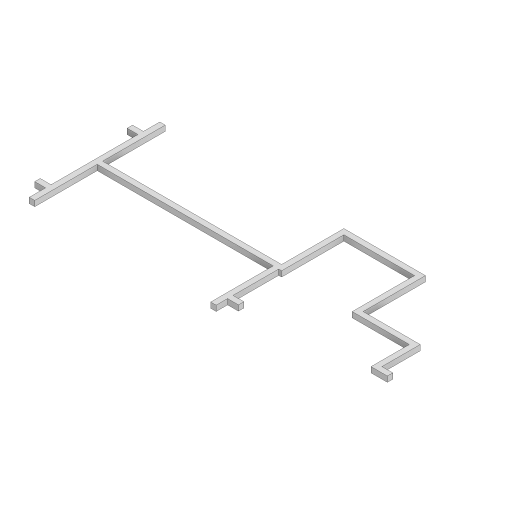
# Autodesk Inventor part: Positioning Stencil
Saved by Autodesk Inventor 2023.4 (Build 274418000, 418)
## iProperties
Created: 2024-03-21
Part Number: Positioning Stencil
Material: Generic
Document SubType Name: Modeling
Designer: josep
Density: 1 g/cm^3
Appearance: Default
Author: josep
Autodesk Inventor part; units mm, degrees
ref_plane "YZ Plane" through (0, 0, 0) normal (1, 0, 0) x (0, 1, 0)
ref_plane "XZ Plane" through (0, 0, 0) normal (0, 1, 0) x (-1, 0, 0)
ref_plane "XY Plane" through (0, 0, 0) normal (0, 0, 1) x (1, 0, 0)
sketch "Sketch1" plane through (0, 0, 0) normal (0, 1, 0) x (-1, 0, 0)
  line L0 (142.3035, 60) -> (-142.3035, 60)
  line L1 (-142.3035, 60) -> (-142.3035, -60)
  line L2 (-142.3035, -60) -> (142.3035, -60)
  line L3 (142.3035, -60) -> (142.3035, 60)
  line L4 (142.3035, 45) -> (122.3035, 45)
  line L5 (122.3035, 45) -> (122.3035, -45)
  line L6 (122.3035, -45) -> (142.3035, -45)
  line L7 (132.3035, 45) -> (132.3035, 40)
  line L8 (132.3035, 40) -> (122.3035, 40)
  line L9 (132.3035, -45) -> (132.3035, -40)
  line L10 (132.3035, -40) -> (122.3035, -40)
  line L11 (122.3035, -45) -> (122.3035, -60)
  line L12 (117.3035, -60) -> (117.3035, -2.5)
  line L13 (117.3035, -2.5) -> (-142.3035, -2.5)
  line L14 (122.3035, 45) -> (122.3035, 60)
  line L15 (117.3035, 60) -> (117.3035, 2.5)
  line L16 (117.3035, 2.5) -> (-142.3035, 2.5)
  line L17 (-169.8065, 2.5) -> (-169.8065, 37.7)
  line L18 (-169.8065, 37.7) -> (-142.3035, 37.7)
  line L19 (-142.3035, 32.7) -> (-174.8065, 32.7)
  line L20 (-174.8065, 32.7) -> (-174.8065, 2.5)
  line L21 (-49.5965, 60) -> (-49.5965, 67.5)
  line L22 (-49.5965, 60) -> (-49.5965, 67.5)
  line L23 (-49.5965, 60) -> (-49.5965, 55.5)
  line L24 (-44.5965, 49.5) -> (-49.5965, 49.5)
  line L25 (-49.5965, 49.5) -> (-49.5965, 55.5)
  line L26 (-44.5965, 29.5) -> (-44.5965, 2.5)
  line L27 (-49.5965, 50.5) -> (-49.5965, 2.5)
  line L28 (-47.3065, -2.5) -> (-47.3065, -39.629)
  line L29 (-117.3065, -39.629) -> (-117.3065, -35.2)
  line L30 (-52.3065, -35.2) -> (-52.3065, -2.5)
  line L31 (-174.8065, 2.5) -> (-174.8065, -2.5)
  line L32 (-117.3065, -35.2) -> (-117.3065, -2.5)
  line L33 (-122.3065, -2.5) -> (-122.3065, -39.629)
  line L34 (-122.3065, -39.629) -> (-117.3065, -39.629)
  line L35 (-117.3065, -2.5) -> (-117.3065, 2.5)
  line L36 (-122.3065, -2.5) -> (-122.3065, 2.5)
  line L37 (-52.3065, -2.5) -> (-52.3065, 2.5)
  line L38 (-47.3065, -39.629) -> (-47.3065, -59.8)
  line L39 (-47.3065, -59.8) -> (-52.3065, -59.8)
  line L40 (-52.3065, -59.8) -> (-52.3065, -35.2)
  line L41 (-52.3065, -59.8) -> (-122.3065, -59.8)
  line L42 (-122.3065, -59.8) -> (-122.3065, -39.629)
  line L43 (-117.3065, -39.629) -> (-117.3065, -59.8)
  line L44 (-52.3065, -54.8) -> (-117.3065, -54.8)
  line L45 (0, -2.5) -> (0, 2.5)
  line L46 (-174.8065, 32.7) -> (-184.8065, 32.7)
  line L47 (-184.8065, 32.7) -> (-184.8065, 37.7)
  line L48 (-184.8065, 37.7) -> (-142.3035, 37.7)
  line L49 (-44.5965, 29.5) -> (-44.5965, 49.5)
  line L50 (-49.5965, 49.9226) -> (-49.5965, 49.5)
  line L51 (-44.5965, 49.5) -> (-44.5965, 64.5)
  line L52 (-44.5965, 64.5) -> (-49.5965, 64.5)
  line L53 (-49.5965, 49.5) -> (-59.5965, 49.5)
  line L54 (-59.5965, 49.5) -> (-59.5965, 44.5)
  line L55 (-59.5965, 44.5) -> (-49.5965, 44.5)
  line L56 (117.3035, -2.5) -> (117.3035, 2.5)
  line L57 (-142.3035, -2.5) -> (-174.8065, -2.5)
  line L58 (-142.3035, 2.5) -> (-169.8065, 2.5)
  point P0 (0, 0)
  point P1 (142.3035, 0)
  point P2 (0, -60)
  point P3 (-158.555, 32.7)
  point P4 (-14.5965, 67.5)
  point P5 (-14.5965, 60)
  point P6 (-159.8035, 32.7)
  point P7 (-44.5965, 60)
  point P8 (-169.8065, 32.7)
  dimension "d0" = 284.607
  dimension "d1" = 120
  dimension "d2" = 15
  dimension "d3" = 15
  dimension "d4" = 10
  dimension "d5" = 5
  dimension "d6" = 5
  dimension "d7" = 5
  dimension "d14" = 0
  dimension "d15" = 0
  dimension "d17" = 12.3
  dimension "d18" = 57.5
  dimension "d19" = 57.5
  dimension "d20" = 5
  dimension "d26" = 171.9
  dimension "d30" = 4.5
  dimension "d34" = 20
  dimension "d36" = 174.61
  dimension "d37" = 5
  dimension "d38" = 5
  dimension "d39" = 65
  dimension "d42" = 9.8
  dimension "d43" = 5
  dimension "d48" = 297.11
  dimension "d49" = 5
  dimension "d50" = 15
  dimension "d51" = 4.5
  dimension "d52" = 5
  dimension "d53" = 5
  dimension "d54" = 15
  dimension "d55" = 10
  constraints: 116 end point, 30 point on line, 20 vertical, 19 perpendicular, 5 horizontal, 5 midpoint, 5 parallel, 3 collinear, 11 other
  measures "d0" distance of L0.start L0.end
  measures "d1" distance of L2.end L0.start
  measures "d2" distance of L4.start L0.start
  measures "d3" distance of L2.end L6.end
  measures "d4" distance of L7.end L8.end
  measures "d5" distance of L7.start L7.end
  measures "d6" distance of L9.start L9.end
  measures "d7" distance between parallel lines of L11 L12
  measures "d14" vertical distance of point (142.304, 0) point (0, 0)
  measures "d15" horizontal distance of point (0, -60) point (0, 0)
  measures "d17" vertical distance of L19.end L4.end
  measures "d18" distance of L15.start L15.end
  measures "d19" distance between parallel lines of L2 L13
  measures "d20" distance from line of point (-158.555, 32.7) L18
  measures "d26" distance of L21.start L14.end
  measures "d30" vertical distance of L14.end L23.end
  measures "d34" distance of L26.start L24.start
  measures "d36" horizontal distance of L5.end L30.start
  measures "d37" distance between parallel lines of L28 L30
  measures "d38" distance between parallel lines of L33 L32
  measures "d39" distance of L29.end L30.start
  measures "d42" vertical distance of L5.end L44.start
  measures "d43" distance between parallel lines of L44 L41
  measures "d48" horizontal distance of L4.end L19.end
  measures "d49" distance between parallel lines of L20 L17
  measures "d50" distance of L47.end L17.end
  measures "d51" vertical distance of L4.end L24.start
  measures "d52" distance of L53.end L54.end
  measures "d53" distance of L51.end L52.end
  measures "d54" distance of L24.start L51.end
  measures "d55" distance of L54.end L55.end
extrude "Extrusion1" add sketch "Sketch1" along normal blind 5 contours L14 L5 L11 L2 L12 L56 L15 L0 | L4 L7 L8 L5 | L51 L24 L25 L23 L0 | L56 L13 L45 L16 | L6 L5 L10 L9 | L49 L26 L16 L27 L24 | L45 L13 L37 L16 | L27 L55 L54 L53 | L28 L38 L39 L40 L30 L13 | L17 L19 L46 L47 L48 | L57 L31 L20 L19 L17 L58 L1 | L1 L16 L36 L13 | L35 L13 L36 L16 | L32 L29 L34 L33 L13 | L40 L41 L43 L44 | L34 L43 L41 L42
body "Solid1"
